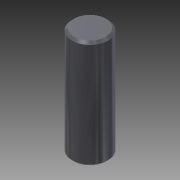
# Autodesk Inventor part: Ax
Saved by Autodesk Inventor 2011 SP2 (Build 150309200, 309)
## iProperties
Created: 2023-03-20
Part Number: Ax
Document SubType Name: Modeling
Designer: utilizator
Density: 1 g/cm^3
Author: utilizator
Autodesk Inventor part; units mm, degrees
ref_plane "YZ Plane" through (0, 0, 0) normal (1, 0, 0) x (0, 1, 0)
ref_plane "XZ Plane" through (0, 0, 0) normal (0, 1, 0) x (-1, 0, 0)
ref_plane "XY Plane" through (0, 0, 0) normal (0, 0, 1) x (1, 0, 0)
sketch "Sketch1" plane through (0, 0, 0) normal (0, 0, 1) x (1, 0, 0)
  line L0 (-11.2, 0) -> (11.2, 0) projected
  line L1 (0, -11.2) -> (0, 11.2) projected
  circle A0 centre (0, 0) radius 8
  dimension "d0" = 8
  constraints: 1 centre point, 1 coincident
  measures "d0" radius of A0
extrude "Extrusion1" add sketch "Sketch1" along normal blind 48
chamfer "Chamfer1" distance 1 angle 45 1 edges at (-8, 0, 48)
chamfer "Chamfer2" distance 1 angle 45 1 edges at (-8, 0, 0)
body "Solid1"
